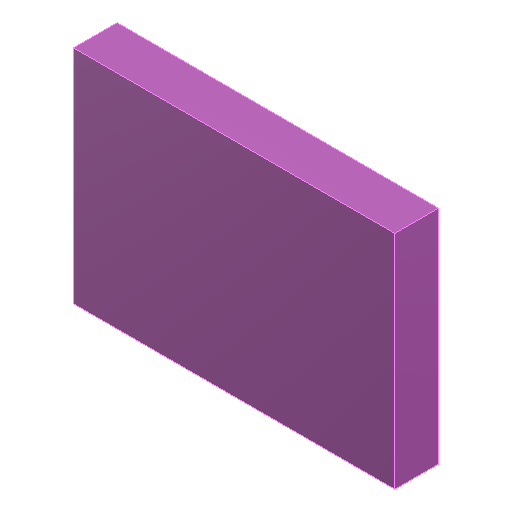
# Autodesk Inventor part: XC1_C050-050X075
Saved by Autodesk Inventor 2022 (Build 260153000, 153)
## iProperties
Created: 2022-01-18
Part Number: XC1_C050-050X075
Material: Generisch
Document SubType Name: Modeling
Designer: diederichbenedict
Density: 1 g/cm^3
Appearance: C050-050X075, XC1_C050-050X075
Author: diederichbenedict
Autodesk Inventor part; units mm, degrees
ref_plane "YZ Plane" through (0, 0, 0) normal (1, 0, 0) x (0, 1, 0)
ref_plane "XZ Plane" through (0, 0, 0) normal (0, 1, 0) x (-1, 0, 0)
ref_plane "XY Plane" through (0, 0, 0) normal (0, 0, 1) x (1, 0, 0)
sketch "C050-050X075, XC1_C050-050X075_11" plane through (0, 0, 0) normal (0, 0, 1) x (1, 0, 0)
  line L0 (-3.683, 2.54) -> (3.683, 2.54)
  line L1 (3.683, 2.54) -> (3.683, -2.54)
  line L2 (3.683, -2.54) -> (-3.683, -2.54)
  line L3 (-3.683, -2.54) -> (-3.683, 2.54)
  constraints: 8 end point
extrude "Extrusion1" add sketch "C050-050X075, XC1_C050-050X075_11" along normal blind 1
